Grundakkus_mit zwischensteg_grob_innen_v4 (Autodesk Fusion 360 design; units mm, degrees)
Autodesk Fusion 360 part; units mm, degrees
sketch "Skizze1" plane through (0, 0, 0) normal (0, 1, 0) x (1, 0, 0)
box "Grundkörper Quader1" add length 51.5 width 42 height 160 placed x (0, 0, -1) y (-1, 0, 0) z (0, 1, 0) at (42, 0, 0) makes body 1
box "Grundkörper Quader3" add length 51.5 width 28 height 160 placed x (0, 0, -1) y (-1, 0, 0) z (0, 1, 0) at (70, 0, 0) separate body makes body 2
copy_body "Körper kopieren/einfügen1" bodies 1 2 makes body 3 makes body 4
move_body "Verschieben1" bodies 3 4 to x (1, 0, 0) y (0, 1, 0) z (0, 0, 1) at (0, 0, -60)
box "Grundkörper Quader5" add length 115.5 width 74 height 160 placed x (0, 0, -1) y (-1, 0, 0) z (0, 1, 0) at (74, 0, 0) separate body makes body 5
move_body "Verschieben2" bodies 5 to x (1, 0, 0) y (0, 1, 0) z (0, 0, 1) at (2, -2, 2)
move_body "Verschieben3" bodies 5 to x (1, 0, 0) y (0, 1, 0) z (0, 0, 1) at (-4, 0, 0)
move_face "Fläche verschieben1" by (2, 0, 0) 1 faces at (72, 51.3333, -75) on bodies 5
move_body "Verschieben4" bodies 2 4 to x (1, 0, 0) y (0, 1, 0) z (0, 0, 1) at (2, 0, 0)
move_face "Fläche verschieben2" by (0, 0, 2.5) 1 faces at (53.3333, 53.3333, -51.5) on bodies 2
move_face "Fläche verschieben3" by (0, 0, 2.5) 1 faces at (53.3333, 53.3333, -111.5) on bodies 4
move_body "Verschieben5" bodies 4 2 to x (1, 0, 0) y (0, 1, 0) z (0, 0, 1) at (0, 0, -1.25)
box "Grundkörper Quader6" add length 43.5 width 2 height 180 placed x (0, 0, -1) y (-1, 0, 0) z (0, 1, 0) at (44, 0, 0) separate body makes body 6
copy_body "Körper kopieren/einfügen2" bodies 6 makes body 7
move_body "Verschieben6" bodies 7 to x (1, 0, 0) y (0, 1, 0) z (0, 0, 1) at (0, 0, -64)
move_body "Verschieben7" bodies 6 to x (1, 0, 0) y (0, 1, 0) z (0, 0, 1) at (0, 0, -4)
combine "Kombinieren1" operation cut target body 5 tool bodies 1 3 4 2 6 7 keep tools result as body 8 in component "Component"
component "Component" placed x (1, 0, 0) y (0, 1, 0) z (0, 0, 1) at (0, 0, 0)
